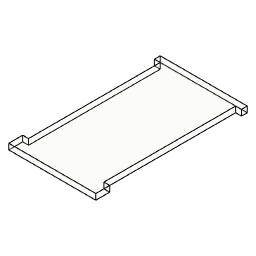
top_plate (Autodesk Fusion 360 design; units mm, degrees)
Autodesk Fusion 360 part; units mm, degrees
sketch "Esquisse1" plane through (0, 0, 0) normal (0, 0, 1) x (1, 0, 0)
  line L0 (75, -125) -> (-75, -125) construction
  line L1 (-75, -125) -> (-75, 125) construction
  line L2 (-75, 125) -> (75, 125) construction
  line L3 (75, 125) -> (75, -125) construction
  line L4 (75, -125) -> (-75, 125) construction
  line L5 (-75, -125) -> (75, 125) construction
  line L6 (-75, 125) -> (75, 125) construction
  line L7 (75, 125) -> (75, 136) construction
  line L8 (75, 136) -> (-75, 136) construction
  line L9 (-75, 136) -> (-75, 125) construction
  line L10 (-75, 136) -> (-75, 126)
  line L11 (-75, 126) -> (-65, 126)
  line L12 (-65, 126) -> (-65, -101)
  line L13 (-65, -101) -> (-75, -101)
  line L14 (-75, -101) -> (-75, -125)
  line L15 (-75, -125) -> (0, -125)
  line L16 (0, -125) -> (0, -120)
  line L17 (0, -120) -> (0, 136)
  line L18 (-75, 136) -> (0, 136)
  line L19 (75, 136) -> (0, 136)
  line L20 (75, 136) -> (75, 125) construction
  line L21 (0, -120) -> (0, 136)
  line L22 (0, -125) -> (0, -120)
  line L23 (75, -101) -> (75, -125)
  line L24 (75, -125) -> (0, -125)
  line L25 (65, -101) -> (75, -101)
  line L26 (75, -125) -> (75, 125) construction
  line L27 (75, 126) -> (65, 126)
  line L28 (75, 136) -> (75, 126)
  line L29 (65, 126) -> (65, -101)
  dimension "d1" = 150
  dimension "d2" = 250
  dimension "d3" = 11
  dimension "d4" = 10
  dimension "d5" = 10
  dimension "d6" = 24
  constraint horizontal L0
  constraint perpendicular L0 L1
  constraint parallel L0 L2
  constraint parallel L1 L3
  constraint coincident L4 origin
  constraint coincident L5 origin
  constraint horizontal L6
  constraint vertical L7
  constraint horizontal L8
  constraint vertical L9
  constraint coincident L9 L10.end
  constraint perpendicular L2 L10
  constraint perpendicular L10 L11
  constraint perpendicular L2 L12
  constraint coincident L1 L13.end
  constraint perpendicular L1 L13
  constraint midpoint L0 L15.end
  constraint perpendicular L0 L16
  constraint midpoint L8 L17.end
  constraint perpendicular L8 L17
  constraint symmetric L0.end L17 L0.start
  constraint symmetric L1.end L17 L2.end
  constraint symmetric L8.end L17 L7.end
  constraint symmetric L10.end L17 L27.start
  constraint symmetric L11.end L17 L27.end
  constraint symmetric L12.end L17 L25.start
  constraint symmetric L13.end L17 L23.start
  constraint symmetric L15.end L17 L16.start
  constraint symmetric L16.end L17 L21.start
  constraint symmetric L18.end L17 L19.end
  measures "d1" distance of L0.start L0.end
  measures "d2" distance of L0.start L2.end
  measures "d3" distance of L1.end L8.end
  measures "d4" distance of L10.end L11.end
  measures "d5" distance of L8 L11
  measures "d6" distance of L13 L15
extrude "Extrusion1" add sketch "Esquisse1" along normal blind 10
